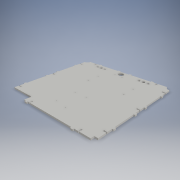
# Autodesk Inventor part: painel inferior
Saved by Autodesk Inventor 2016 (Build 200138000, 138)
## iProperties
Created: 2016-08-08
Part Number: painel inferior
Material: Generic
Document SubType Name: Modeling
Designer: Waldo
Density: 1 g/cm^3
Appearance: Default
Author: Waldo
Autodesk Inventor part; units mm, degrees
ref_plane "YZ Plane" through (0, 0, 0) normal (1, 0, 0) x (0, 1, 0)
ref_plane "XZ Plane" through (0, 0, 0) normal (0, 1, 0) x (-1, 0, 0)
ref_plane "XY Plane" through (0, 0, 0) normal (0, 0, 1) x (1, 0, 0)
sketch "Sketch1" plane through (0, 0, 0) normal (0, 1, 0) x (-1, 0, 0)
  line L0 (95, 0) -> (102.5, 0)
  line L1 (95, 0) -> (95, -25)
  line L2 (95, -25) -> (0, -25)
  line L3 (0, -41.36) -> (0, -25)
  line L4 (6.5002, -41.36) -> (0, -41.36)
  line L5 (9.5783, -40.0697) -> (8.0283, -40.0697)
  line L6 (10.8802, -40.9478) -> (10.8802, -40.7785)
  line L7 (10.8802, -45.0415) -> (10.8802, -44.8722)
  line L8 (8.0283, -45.7503) -> (9.5783, -45.7503)
  line L9 (0, -44.46) -> (6.5002, -44.46)
  line L10 (0, -62.8) -> (0, -44.46)
  line L11 (-4.5, -62.8) -> (0, -62.8)
  line L12 (-4.5, -72.8) -> (-4.5, -62.8)
  line L13 (0, -72.8) -> (-4.5, -72.8)
  line L14 (0, -153.5) -> (0, -72.8)
  line L15 (-4.5, -153.5) -> (0, -153.5)
  line L16 (-4.5, -163.5) -> (-4.5, -153.5)
  line L17 (0, -163.5) -> (-4.5, -163.5)
  line L18 (0, -181.8556) -> (0, -163.5)
  line L19 (6.5002, -181.8556) -> (0, -181.8556)
  line L20 (9.5783, -180.5653) -> (8.0283, -180.5653)
  line L21 (10.8802, -181.4434) -> (10.8802, -181.2741)
  line L22 (10.8802, -185.5371) -> (10.8802, -185.3679)
  line L23 (8.0283, -186.246) -> (9.5783, -186.246)
  line L24 (0, -184.9556) -> (6.5002, -184.9556)
  line L25 (0, -203.5) -> (0, -184.9556)
  line L26 (-4.5, -203.5) -> (0, -203.5)
  line L27 (-4.5, -213.5) -> (-4.5, -203.5)
  line L28 (0, -213.5) -> (-4.5, -213.5)
  line L29 (0, -294.2) -> (0, -213.5)
  line L30 (-4.5, -294.2) -> (0, -294.2)
  line L31 (-4.5, -304.2) -> (-4.5, -294.2)
  line L32 (0, -304.2) -> (-4.5, -304.2)
  line L33 (0, -322.2809) -> (0, -304.2)
  line L34 (6.5002, -322.2809) -> (0, -322.2809)
  line L35 (10.2574, -321.1473) -> (8.7074, -321.1473)
  line L36 (10.8802, -321.8687) -> (10.8802, -321.6994)
  line L37 (10.8802, -326.1191) -> (10.8802, -326.1066)
  line L38 (8.0283, -326.828) -> (9.5783, -326.828)
  line L39 (0, -325.5376) -> (6.5002, -325.5376)
  line L40 (0, -350.5) -> (0, -325.5376)
  line L41 (50.0981, -367) -> (16.5, -367)
  line L42 (50.0981, -360.4998) -> (50.0981, -367)
  line L43 (48.8078, -357.4217) -> (48.8078, -358.9717)
  line L44 (49.6859, -356.1198) -> (49.5166, -356.1198)
  line L45 (53.7796, -356.1198) -> (53.6104, -356.1198)
  line L46 (54.4885, -358.9717) -> (54.4885, -357.4217)
  line L47 (53.1981, -367) -> (53.1981, -360.4998)
  line L48 (67.5, -367) -> (53.1981, -367)
  line L49 (67.5, -371.5) -> (67.5, -367)
  line L50 (77.5, -371.5) -> (67.5, -371.5)
  line L51 (77.5, -367) -> (77.5, -371.5)
  line L52 (158, -367) -> (77.5, -367)
  line L53 (158, -371.5) -> (158, -367)
  line L54 (168, -371.5) -> (158, -371.5)
  line L55 (168, -367) -> (168, -371.5)
  line L56 (208, -367) -> (168, -367)
  line L57 (208, -371.5) -> (208, -367)
  line L58 (218, -371.5) -> (208, -371.5)
  line L59 (218, -367) -> (218, -371.5)
  line L60 (298.5, -367) -> (218, -367)
  line L61 (298.5, -371.5) -> (298.5, -367)
  line L62 (308.5, -371.5) -> (298.5, -371.5)
  line L63 (308.5, -367) -> (308.5, -371.5)
  line L64 (322.8019, -367) -> (308.5, -367)
  line L65 (322.8019, -360.4998) -> (322.8019, -367)
  line L66 (321.5115, -357.4217) -> (321.5115, -358.9717)
  line L67 (322.3896, -356.1198) -> (322.2204, -356.1198)
  line L68 (326.4834, -356.1198) -> (326.3141, -356.1198)
  line L69 (327.1922, -358.9717) -> (327.1922, -357.4217)
  line L70 (325.9019, -367) -> (325.9019, -360.4998)
  line L71 (359.5, -367) -> (325.9019, -367)
  line L72 (376, -325.278) -> (376, -350.5)
  line L73 (369.4998, -325.278) -> (376, -325.278)
  line L74 (366.4217, -326.5683) -> (367.9717, -326.5683)
  line L75 (365.1198, -325.6902) -> (365.1198, -325.8594)
  line L76 (365.1198, -321.5965) -> (365.1198, -321.7657)
  line L77 (367.9717, -320.8876) -> (366.4217, -320.8876)
  line L78 (376, -322.178) -> (369.4998, -322.178)
  line L79 (376, -304.2) -> (376, -322.178)
  line L80 (380.5, -304.2) -> (376, -304.2)
  line L81 (380.5, -294.2) -> (380.5, -304.2)
  line L82 (376, -294.2) -> (380.5, -294.2)
  line L83 (376, -213.5) -> (376, -294.2)
  line L84 (380.5, -213.5) -> (376, -213.5)
  line L85 (380.5, -203.5) -> (380.5, -213.5)
  line L86 (376, -203.5) -> (380.5, -203.5)
  line L87 (376, -184.7911) -> (376, -203.5)
  line L88 (369.4998, -184.7911) -> (376, -184.7911)
  line L89 (366.4217, -186.0814) -> (367.9717, -186.0814)
  line L90 (365.1198, -185.2033) -> (365.1198, -185.3726)
  line L91 (365.1198, -181.1096) -> (365.1198, -181.2788)
  line L92 (367.9717, -180.4008) -> (366.4217, -180.4008)
  line L93 (376, -181.6911) -> (369.4998, -181.6911)
  line L94 (376, -163.5) -> (376, -181.6911)
  line L95 (380.5, -163.5) -> (376, -163.5)
  line L96 (380.5, -153.5) -> (380.5, -163.5)
  line L97 (376, -153.5) -> (380.5, -153.5)
  line L98 (376, -72.8) -> (376, -153.5)
  line L99 (380.5, -72.8) -> (376, -72.8)
  line L100 (380.5, -62.8) -> (380.5, -72.8)
  line L101 (376, -62.8) -> (380.5, -62.8)
  line L102 (376, -44.2864) -> (376, -62.8)
  line L103 (369.4998, -44.2864) -> (376, -44.2864)
  line L104 (366.4217, -45.5768) -> (367.9717, -45.5768)
  line L105 (365.1198, -44.6987) -> (365.1198, -44.8679)
  line L106 (365.1198, -40.6049) -> (365.1198, -40.7742)
  line L107 (367.9717, -39.8961) -> (366.4217, -39.8961)
  line L108 (376, -41.1864) -> (369.4998, -41.1864)
  line L109 (376, -12) -> (376, -41.1864)
  line L110 (364, -12) -> (376, -12)
  line L111 (364, 0) -> (364, -12)
  line L112 (325.9019, 0) -> (364, 0)
  line L113 (325.9019, -6.5002) -> (325.9019, 0)
  line L114 (327.1922, -9.5783) -> (327.1922, -8.0283)
  line L115 (326.3141, -10.8802) -> (326.4834, -10.8802)
  line L116 (322.2204, -10.8802) -> (322.3896, -10.8802)
  line L117 (321.5115, -8.0283) -> (321.5115, -9.5783)
  line L118 (322.8019, 0) -> (322.8019, -6.5002)
  line L119 (308.5, 0) -> (322.8019, 0)
  line L120 (308.5, 4.5) -> (308.5, 0)
  line L121 (298.5, 4.5) -> (308.5, 4.5)
  line L122 (298.5, 0) -> (298.5, 4.5)
  line L123 (122.5507, 0) -> (298.5, 0)
  line L124 (122.5507, -6.5002) -> (122.5507, 0)
  line L125 (123.841, -9.5783) -> (123.841, -8.0283)
  line L126 (122.9629, -10.8802) -> (123.1322, -10.8802)
  line L127 (118.8692, -10.8802) -> (119.0384, -10.8802)
  line L128 (118.1603, -8.0283) -> (118.1603, -9.5783)
  line L129 (119.4507, 0) -> (119.4507, -6.5002)
  line L130 (112.5, 0) -> (119.4507, 0)
  line L131 (112.5, 4.5) -> (112.5, 0)
  line L132 (102.5, 4.5) -> (112.5, 4.5)
  line L133 (102.5, 0) -> (102.5, 4.5)
  circle A0 centre (301, -346) radius 4.5
  circle A1 centre (265, -346) radius 4.5
  circle A2 centre (75, -346) radius 4.5
  circle A3 centre (111, -346) radius 4.5
  circle A4 centre (188, -346) radius 11
  circle A5 centre (170.2736, -59.9894) radius 1.5
  circle A6 centre (218.2736, -52.4894) radius 1.5
  circle A7 centre (170.2736, -134.9894) radius 1.5
  circle A8 centre (287.7441, -278.3503) radius 2
  circle A9 centre (287.7441, -228.3503) radius 2
  circle A10 centre (137.7441, -228.3503) radius 2
  circle A11 centre (137.7441, -278.3503) radius 2
  circle A12 centre (218.2736, -134.9894) radius 1.5
  circle A13 centre (283, -346) radius 6
  circle A14 centre (93, -346) radius 6
  circle A15 centre (172.5, -330.5) radius 1.6
  circle A16 centre (203.5, -330.5) radius 1.6
  circle A17 centre (203.5, -361.5) radius 1.6
  circle A18 centre (172.5, -361.5) radius 1.6
  arc A19 (8.0283, -40.0697) -> (6.5002, -41.36) centre (8.0283, -41.6197) ccw
  arc A20 (10.8802, -40.7785) -> (9.5783, -40.0697) centre (9.5783, -41.6197) ccw
  arc A21 (10.8802, -44.8722) -> (10.8802, -40.9478) centre (8.9187, -42.91) ccw
  arc A22 (9.5783, -45.7503) -> (10.8802, -45.0415) centre (9.5783, -44.2003) ccw
  arc A23 (6.5002, -44.46) -> (8.0283, -45.7503) centre (8.0283, -44.2003) ccw
  arc A24 (8.0283, -180.5653) -> (6.5002, -181.8556) centre (8.0283, -182.1153) ccw
  arc A25 (10.8802, -181.2741) -> (9.5783, -180.5653) centre (9.5783, -182.1153) ccw
  arc A26 (10.8802, -185.3679) -> (10.8802, -181.4434) centre (8.9187, -183.4056) ccw
  arc A27 (9.5783, -186.246) -> (10.8802, -185.5371) centre (9.5783, -184.696) ccw
  arc A28 (6.5002, -184.9556) -> (8.0283, -186.246) centre (8.0283, -184.696) ccw
  arc A29 (8.7074, -321.1473) -> (6.5002, -322.2809) centre (8.0283, -322.5406) ccw
  arc A30 (10.8802, -321.6994) -> (10.2574, -321.1473) centre (9.5783, -322.5406) ccw
  arc A31 (10.8802, -326.1066) -> (10.8802, -321.8687) centre (8.9187, -323.9876) ccw
  arc A32 (9.5783, -326.828) -> (10.8802, -326.1191) centre (9.5783, -325.278) ccw
  arc A33 (6.5002, -325.5376) -> (8.0283, -326.828) centre (8.0283, -325.278) ccw
  arc A34 (16.5, -367) -> (0, -350.5) centre (0, -367) ccw
  arc A35 (48.8078, -358.9717) -> (50.0981, -360.4998) centre (50.3578, -358.9717) ccw
  arc A36 (49.5166, -356.1198) -> (48.8078, -357.4217) centre (50.3578, -357.4217) ccw
  arc A37 (53.6104, -356.1198) -> (49.6859, -356.1198) centre (51.6481, -358.0813) ccw
  arc A38 (54.4885, -357.4217) -> (53.7796, -356.1198) centre (52.9385, -357.4217) ccw
  arc A39 (53.1981, -360.4998) -> (54.4885, -358.9717) centre (52.9385, -358.9717) ccw
  arc A40 (321.5115, -358.9717) -> (322.8019, -360.4998) centre (323.0615, -358.9717) ccw
  arc A41 (322.2204, -356.1198) -> (321.5115, -357.4217) centre (323.0615, -357.4217) ccw
  arc A42 (326.3141, -356.1198) -> (322.3896, -356.1198) centre (324.3519, -358.0813) ccw
  arc A43 (327.1922, -357.4217) -> (326.4834, -356.1198) centre (325.6422, -357.4217) ccw
  arc A44 (325.9019, -360.4998) -> (327.1922, -358.9717) centre (325.6422, -358.9717) ccw
  arc A45 (376, -350.5) -> (359.5, -367) centre (376, -367) ccw
  arc A46 (367.9717, -326.5683) -> (369.4998, -325.278) centre (367.9717, -325.0183) ccw
  arc A47 (365.1198, -325.8594) -> (366.4217, -326.5683) centre (366.4217, -325.0183) ccw
  arc A48 (365.1198, -321.7657) -> (365.1198, -325.6902) centre (367.0813, -323.728) ccw
  arc A49 (366.4217, -320.8876) -> (365.1198, -321.5965) centre (366.4217, -322.4376) ccw
  arc A50 (369.4998, -322.178) -> (367.9717, -320.8876) centre (367.9717, -322.4376) ccw
  arc A51 (367.9717, -186.0814) -> (369.4998, -184.7911) centre (367.9717, -184.5314) ccw
  arc A52 (365.1198, -185.3726) -> (366.4217, -186.0814) centre (366.4217, -184.5314) ccw
  arc A53 (365.1198, -181.2788) -> (365.1198, -185.2033) centre (367.0813, -183.2411) ccw
  arc A54 (366.4217, -180.4008) -> (365.1198, -181.1096) centre (366.4217, -181.9508) ccw
  arc A55 (369.4998, -181.6911) -> (367.9717, -180.4008) centre (367.9717, -181.9508) ccw
  arc A56 (367.9717, -45.5768) -> (369.4998, -44.2864) centre (367.9717, -44.0268) ccw
  arc A57 (365.1198, -44.8679) -> (366.4217, -45.5768) centre (366.4217, -44.0268) ccw
  arc A58 (365.1198, -40.7742) -> (365.1198, -44.6987) centre (367.0813, -42.7364) ccw
  arc A59 (366.4217, -39.8961) -> (365.1198, -40.6049) centre (366.4217, -41.4461) ccw
  arc A60 (369.4998, -41.1864) -> (367.9717, -39.8961) centre (367.9717, -41.4461) ccw
  arc A61 (327.1922, -8.0283) -> (325.9019, -6.5002) centre (325.6422, -8.0283) ccw
  arc A62 (326.4834, -10.8802) -> (327.1922, -9.5783) centre (325.6422, -9.5783) ccw
  arc A63 (322.3896, -10.8802) -> (326.3141, -10.8802) centre (324.3519, -8.9187) ccw
  arc A64 (321.5115, -9.5783) -> (322.2204, -10.8802) centre (323.0615, -9.5783) ccw
  arc A65 (322.8019, -6.5002) -> (321.5115, -8.0283) centre (323.0615, -8.0283) ccw
  arc A66 (123.841, -8.0283) -> (122.5507, -6.5002) centre (122.291, -8.0283) ccw
  arc A67 (123.1322, -10.8802) -> (123.841, -9.5783) centre (122.291, -9.5783) ccw
  arc A68 (119.0384, -10.8802) -> (122.9629, -10.8802) centre (121.0007, -8.9187) ccw
  arc A69 (118.1603, -9.5783) -> (118.8692, -10.8802) centre (119.7103, -9.5783) ccw
  arc A70 (119.4507, -6.5002) -> (118.1603, -8.0283) centre (119.7103, -8.0283) ccw
  circle A71 centre (111, -346) radius 1.5
  circle A72 centre (75, -346) radius 1.5
  circle A73 centre (265, -346) radius 1.5
  circle A74 centre (301, -346) radius 1.5
  circle A75 centre (188, -346) radius 7
  point P0 (0, 0)
  constraints: 268 end point, 104 point on circle, 97 parallel, 76 centre point, 65 equal radius, 43 tangent, 30 perpendicular, 4 collinear
extrude "Extrusion1" add sketch "Sketch1" along normal blind 6 contours L0 L133 L132 L131 L130 L129 A70 L128 A69 L127 A68 L126 A67 L125 A66 L124 L123 L122 L121 L120 L119 L118 A65 L117 A64 L116 A63 L115 A62 L114 A61 L113 L112 L111 L110 L109 L108 A60 L107 A59 L106 A58 L105 A57 L104 A56 L103 L102 L101 L100 L99 L98 L97 L96 L95 L94 L93 A55 L92 A54 L91 A53 L90 A52 L89 A51 L88 L87 L86 L85 L84 L83 L82 L81 L80 L79 L78 A50 L77 A49 L76 A48 L75 A47 L74 A46 L73 L72 A45 L71 L70 A44 L69 A43 L68 A42 L67 A41 L66 A40 L65 L64 L63 L62 L61 L60 L59 L58 L57 L56 L55 L54 L53 L52 L51 L50 L49 L48 L47 A39 L46 A38 L45 A37 L44 A36 L43 A35 L42 L41 A34 L40 L39 A33 L38 A32 L37 A31 L36 A30 L35 A29 L34 L33 L32 L31 L30 L29 L28 L27 L26 L25 L24 A28 L23 A27 L22 A26 L21 A25 L20 A24 L19 L18 L17 L16 L15 L14 L13 L12 L11 L10 L9 A23 L8 A22 L7 A21 L6 A20 L5 A19 L4 L3 L2 L1
body "Solid1"
